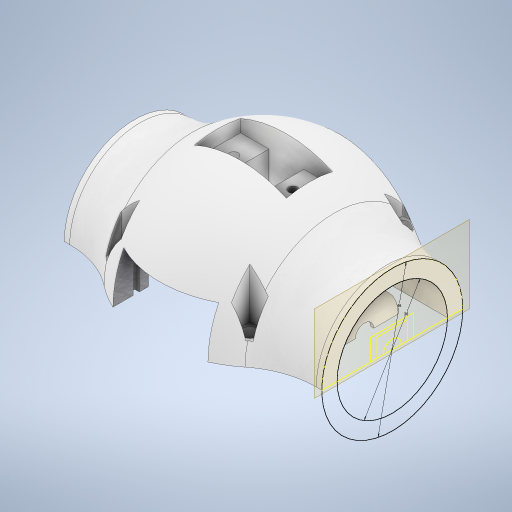
# Autodesk Inventor part: body front moter middle lemon shape
Saved by Autodesk Inventor 2023 (Build 270158000, 158)
## iProperties
Created: 2022-10-08
Part Number: body front moter middle lemon shape
Material: ABS プラスチック
Document SubType Name: Modeling
Designer: ellie
Density: 1.06 g/cm^3
Appearance: 積雪
Author: ellie
Autodesk Inventor part; units mm, degrees
ref_plane "YZ Plane" through (0, 0, 0) normal (1, 0, 0) x (0, 1, 0)
ref_plane "XZ Plane" through (0, 0, 0) normal (0, 1, 0) x (-1, 0, 0)
ref_plane "XY Plane" through (0, 0, 0) normal (0, 0, 1) x (1, 0, 0)
sketch "スケッチ1" plane through (0, 0, 0) normal (0, 1, 0) x (-1, 0, 0)
  circle A0 centre (0, 0) radius 37
  line L0 (0, 0) -> (0, -37)
  line L1 (0, 0) -> (0, 37)
  dimension "d0" = 74
  constraints: 4 end point, 2 point on circle, 2 vertical, 1 centre point, 1 coincident
  measures "d0" diameter of A0
revolve "回転1" add sketch "スケッチ1" angle 180 about axis through (0, 0, 0) along (0, 0, 1) picked at (-2.7444, -24.3574) contours L1 L0 A0
sketch "スケッチ5" plane through (0, 0, 0) normal (0, -1, 0) x (1, 0, 0)
  line L0 (-20, -21) -> (20, -21)
  line L1 (20, -21) -> (20, -11)
  line L2 (20, -11) -> (-20, -11)
  line L3 (-20, -11) -> (-20, -21)
  line L4 (-20, -13) -> (-20, -11)
  line L5 (0, 27) -> (-17, 27)
  line L6 (-17, 27) -> (-17, 25)
  line L7 (-17, 25) -> (0, 25)
  line L8 (0, 25) -> (0, 27)
  line L9 (0, 22) -> (-20, 22)
  line L10 (-20, 22) -> (-20, 21)
  line L11 (-20, 21) -> (0, 21)
  line L12 (0, 21) -> (0, 22)
  line L13 (0, 15) -> (-21, 15)
  line L14 (-21, 15) -> (-21, 13)
  line L15 (-21, 13) -> (0, 13)
  line L16 (0, 13) -> (0, 15)
  line L17 (0, 7) -> (-23, 7)
  line L18 (-23, 7) -> (-23, 5)
  line L19 (-23, 5) -> (0, 5)
  line L20 (0, 5) -> (0, 7)
  circle A0 centre (0, 0) radius 37 projected
  circle A1 centre (0, 0) radius 37 projected
  line L21 (0, 37) -> (0, -37)
  line L22 (37, 0) -> (-37, 0)
  line L23 (-32, 5) -> (-23, 5)
  line L24 (-23, 5) -> (-23, -5)
  line L25 (-23, -5) -> (-32, -5)
  line L26 (-32, -5) -> (-32, 5)
  line L27 (-23, -8.0262) -> (-23, 5)
  line L28 (-29, 22.9783) -> (-29, -22.9783)
  line L29 (-15.5, 27) -> (0, 27)
  line L30 (0, 27) -> (0, 37)
  line L31 (0, 37) -> (-15.5, 37)
  line L32 (-15.5, 37) -> (-15.5, 27)
  line L33 (-15.5, 25) -> (0, 25)
  line L34 (0, 25) -> (0, 22)
  line L35 (0, 22) -> (-15.5, 22)
  line L36 (-15.5, 22) -> (-15.5, 25)
  line L37 (-19, 15) -> (0, 15)
  line L38 (0, 15) -> (0, 21)
  line L39 (0, 21) -> (-19, 21)
  line L40 (-19, 21) -> (-19, 15)
  line L41 (-19, 13) -> (0, 13)
  line L42 (0, 13) -> (0, 7)
  line L43 (0, 7) -> (-19, 7)
  line L44 (-19, 7) -> (-19, 13)
  line L45 (-23, 0) -> (-39.6865, 0)
  line L46 (-23, 0) -> (-7.8337, 0)
  line L47 (-8, 5) -> (-23, 5)
  line L48 (-23, 5) -> (-23, -5)
  line L49 (-23, -5) -> (-8, -5)
  line L50 (-8, -5) -> (-8, 5)
  line L51 (-8, 5) -> (-23, -5) construction
  line L52 (-23, 5) -> (-8, -5) construction
  line L53 (-23, 7) -> (-33, 7)
  line L54 (-33, 7) -> (-33, -7)
  line L55 (-33, -7) -> (-23, -7)
  line L56 (-23, -7) -> (-23, 7)
  line L57 (-23, 7) -> (-33, -7) construction
  line L58 (-33, 7) -> (-23, -7) construction
  line L59 (-8, 5) -> (-1, 5)
  line L60 (-1, 5) -> (-1, -5)
  line L61 (-1, -5) -> (-8, -5)
  line L62 (-8, -5) -> (-8, 5)
  line L63 (-8, 5) -> (-1, -5) construction
  line L64 (-1, 5) -> (-8, -5) construction
  line L65 (-23, 5) -> (-29, 5)
  line L66 (-23, -5) -> (-29, -5)
  line L67 (-23, 7) -> (-29, 7)
  line L68 (-23, -7) -> (-29, -7)
  line L69 (27.2764, -25) -> (-27.2764, -25)
  line L70 (-8, 5) -> (-6.8, 5)
  line L71 (-6.8, 5) -> (-6.8, -5)
  line L72 (-6.8, -5) -> (-8, -5)
  line L73 (-8, -5) -> (-8, 5)
  line L74 (0, 7) -> (2, 7)
  line L75 (0, -3) -> (0, 7)
  line L76 (-11.5791, -11) -> (-8, -11)
  point P0 (0, -21)
  point P1 (0, -11)
  point P2 (0, 26)
  point P3 (0, 21.5)
  point P4 (0, 14)
  point P5 (0, 6)
  point P6 (-20, -16)
  point P7 (-27, -0.5262)
  point P8 (-29, 22.9783)
  point P9 (-29, -22.9783)
  point P10 (-29, -5)
  point P11 (-15.5, 23.5)
  point P12 (-15.5, 33.5969)
  point P13 (0, 27)
  point P14 (0, 37)
  point P15 (0, 25)
  point P16 (0, 13)
  point P17 (0, 15)
  point P18 (-29, 0)
  point P19 (-32, 0)
  point P20 (-23, 0)
  point P21 (-15.5, 0)
  point P22 (-28, 0)
  point P23 (-4.5, 0)
  point P24 (-8, -5)
  point P25 (-8, 5)
  point P26 (-27, 0.5)
  point P27 (-28, 0.4738)
  point P28 (-28, -11.5262)
  point P29 (-27, -11.5)
  point P30 (-23, 5)
  point P31 (-23, 5)
  point P32 (-23, 5)
  point P33 (-8, 0)
  point P34 (-1, 0)
  point P35 (0, 7)
  point P36 (0, 5)
  point P37 (-29, 7)
  dimension "d12" = 40
  dimension "d13" = 10
  dimension "d23" = 17
  dimension "d24" = 2
  dimension "d27" = 20
  dimension "d28" = 1
  dimension "d30" = 21
  dimension "d31" = 2
  dimension "d33" = 2
  dimension "d88" = 0
  dimension "d89" = 0
  dimension "d90" = 16
  dimension "d92" = 20
  dimension "d93" = 10
  dimension "d97" = 9
  dimension "d98" = 10
  dimension "d113" = 29
  dimension "d122" = 15.5
  dimension "d123" = 37
  dimension "d124" = 3
  dimension "d125" = 15.5
  dimension "d126" = 6
  dimension "d127" = 6
  dimension "d147" = 10
  dimension "d149" = 8
  dimension "d151" = 15
  dimension "d161" = 14
  dimension "d162" = 10
  dimension "d164" = 10
  dimension "d165" = 7
  dimension "d170" = 25
  dimension "d175" = 1.2
  dimension "d187" = 1
  dimension "d262" = 2
  dimension "d263" = 2
  constraints: 152 end point, 29 parallel, 19 horizontal, 17 perpendicular, 15 midpoint, 15 point on line, 9 collinear, 1 vertical, 20 other
  measures "d12" distance of L2.end L1.end
  measures "d13" distance of L1.end L0.end
  measures "d23" distance of L7.end L6.end
  measures "d24" distance of L6.end L5.end
  measures "d27" distance of L11.end L10.end
  measures "d28" distance of L10.end L9.end
  measures "d30" distance of L15.end L14.end
  measures "d31" distance of L14.end L13.end
  measures "d33" distance of L18.end L17.end
  measures "d89" distance from line of point (0, 0) L22
  measures "d90" distance from line of L0 point (0, -37)
  measures "d92" distance of the line from the sketch origin of L3
  measures "d93" distance from line of L5 point (0, 37)
  measures "d97" distance of L24.end L25.end
  measures "d98" distance of L23.end L24.end
  measures "d113" distance of the line from the sketch origin of L28
  measures "d122" distance of the line from the sketch origin of L32
  measures "d123" distance between parallel lines of L31 L22
  measures "d124" distance of L33.end L34.end
  measures "d126" distance of L38.end L37.end
  measures "d127" distance of L41.end L42.end
  measures "d147" distance of L48.end L47.end
  measures "d149" distance of the line from the sketch origin of L50
  measures "d151" distance between parallel lines of L50 L24
  measures "d161" distance between parallel lines of L55 L53
  measures "d162" distance between parallel lines of L48 L54
  measures "d164" distance between parallel lines of L61 L59
  measures "d165" distance between parallel lines of L50 L60
  measures "d170" distance between parallel lines of L69 L22
  measures "d175" distance of L71.end L72.end
  measures "d187" distance between parallel lines of L75 L60
  measures "d262" distance between parallel lines of L14 L44
  measures "d263" distance between parallel lines of L14 L40
extrude "GNSボード" cut sketch "スケッチ5" against normal blind 16 contours L8 L7 L6 L5
extrude "GNSボード止めるよう" cut sketch "スケッチ5" against normal blind 15 contours L21 L5 L32 A0 | L21 L9 L36 L7
extrude "アルミ板１" cut sketch "スケッチ5" against normal blind 20 contours L12 L11 L10 L9
extrude "メイン基板" cut sketch "スケッチ5" against normal blind 21 contours L15 L14 L13 L16
extrude "メイン止めるよう" cut sketch "スケッチ5" against normal blind 16.5 contours L17 L44 L15 L21 | L13 L40 L11 L21
extrude "アルミ板２" cut sketch "スケッチ5" against normal blind 20 contours L19 L18 L17 L20
extrude "電池ボックス入れ" cut sketch "スケッチ5" against normal blind 13 contours L3 L2 L21 L0 | L21 L2 L1 L0
extrude "side ut" cut sketch "スケッチ5" against normal blind 100 contours A0 L22 L54 L55 L28 | A0 L28 L53 L54 L22 | L55 L54 L22 L26 L25 L28 | L54 L53 L28 L23 L26 L22 | L25 L26 L22 L28 | L26 L23 L28 L22
extrude "motor case" add sketch "スケッチ5" against normal blind 7 contours L55 L54 L22 L26 L25 L28 | L28 L25 L27 L55 | L54 L53 L28 L23 L26 L22 | L28 L22 L24 L25 | L25 L26 L22 L28 | L53 L18 L23 L28 | L26 L23 L28 L22 | L24 L22 L50 L49 | L28 L23 L24 L22 | L50 L22 L24 L19
extrude "bottom cut" cut sketch "スケッチ5" against normal blind 90 contours L69 A0 L21 | L21 A0 L69
extrude "motor" cut sketch "スケッチ5" against normal blind 6 contours L60 L61 L71 L22 | L22 L71 L19 L60 | L71 L61 L50 L22 | L22 L50 L19 L71 | L28 L22 L24 L25 | L25 L26 L22 L28 | L26 L23 L28 L22 | L24 L22 L50 L49 | L28 L23 L24 L22 | L50 L22 L24 L19
extrude "motor block" add sketch "スケッチ5" against normal blind 10 contours L71 L61 L50 L22 | L22 L50 L19 L71
sketch "スケッチ26" plane through (-33, 0, -7) normal (-1, 0, 0) x (0, 0, 1)
  line L0 (14, 0) -> (0, 0) projected
  circle A0 centre (7, 0) radius 3
  point P0 (7, 0)
  point P1 (7, 0)
  point P2 (7, 0)
  point P3 (7, 0)
  point P4 (4, 0)
  point P5 (10, 0)
  dimension "d197" = 6
  constraints: 1 centre point, 1 coincident
  measures "d197" diameter of A0
extrude "押し出し34" cut sketch "スケッチ26" against normal blind 27 contours L0 A0 picked at (7.7485, 0.6631)
mirror "ミラー11" about plane through (0, 0, 0) normal (1, 0, 0) of "GNSボード", "GNSボード止めるよう", "アルミ板１", "メイン止めるよう", "メイン基板", "アルミ板２", "motor", "押し出し34", "motor case", "電池ボックス入れ", "motor block", "side ut"
ref_plane "作業平面5" through (0, 13, 0) normal (0, -1, 0) x (1, 0, 0)
ref_plane "作業平面6" through (-15.5, 37, 27) normal (0, -1, 0) x (1, 0, 0)
sketch "スケッチ29" plane through (-15.5, 37, 27) normal (0, -1, 0) x (1, 0, 0)
  line L0 (15.5, -27) -> (-67.7134, -27)
  line L1 (-67.7134, -27) -> (15.5, -27)
  line L2 (110.7852, -24.5555) -> (110.7852, -27.3413)
  line L3 (15.5, -27) -> (98.1975, -27)
  circle A0 centre (25.2, -27) radius 1.5
  circle A1 centre (5.8, -27) radius 1.5
  line L4 (32.5, 0) -> (-1.5, 0) projected
  line L5 (15.5, 0) -> (15.5, -52)
  line L6 (-11.7764, -52) -> (42.7764, -52) projected
  point P0 (-11.5, -52)
  point P1 (42.5, -52)
  dimension "d205" = 3
  dimension "d206" = 19.4
  dimension "d207" = 0
  constraints: 10 end point, 2 centre point, 2 horizontal, 2 midpoint, 1 collinear, 1 vertical, 1 other
  measures "d205" diameter of A0
  measures "d206" distance of A1.centre A0.centre
  measures "d207" distance from line of L3 A0.centre
extrude "押し出し36" cut sketch "スケッチ29" along normal blind 25
sketch "スケッチ30" plane through (-15.5, 37, 27) normal (0, -1, 0) x (1, 0, 0)
  line L0 (0.5, -19.5) -> (30.5, -19.5)
  line L1 (30.5, -19.5) -> (30.5, -34.5)
  line L2 (30.5, -34.5) -> (0.5, -34.5)
  line L3 (0.5, -34.5) -> (0.5, -19.5)
  line L4 (0.5, -19.5) -> (30.5, -34.5) construction
  line L5 (30.5, -19.5) -> (0.5, -34.5) construction
  point P0 (15.5, -27)
  dimension "d210" = 30
  dimension "d211" = 15
  constraints: 12 end point, 2 midpoint, 2 parallel, 1 horizontal, 1 perpendicular
  measures "d210" distance of L1.end L2.end
  measures "d211" distance of L0.end L1.end
extrude "押し出し37" cut sketch "スケッチ30" along normal blind 8
ref_plane "作業平面7" through (-15.5, 12, 27) normal (0, 1, 0) x (1, 0, 0)
sketch "スケッチ33" plane through (-15.5, 12, 27) normal (0, 1, 0) x (1, 0, 0)
  circle A0 centre (25.2, 27) radius 1.5 projected
  circle A1 centre (5.8, 27) radius 1.5 projected
  line L0 (0.5, 34.5) -> (0.5, 19.5) projected
  line L1 (30.5, 19.5) -> (30.5, 34.5) projected
  line L2 (0.5, 19.5) -> (30.5, 19.5) projected
  line L3 (30.5, 34.5) -> (0.5, 34.5) projected
  line L4 (15.5, 0) -> (15.5, 52) projected
  line L5 (15.5, 27) -> (98.1975, 27) projected
  circle A2 centre (25.2, 27) radius 3
  circle A3 centre (5.8, 27) radius 3
  dimension "d219" = 6
  dimension "d220" = 6
  constraints: 2 centre point, 2 coincident
  measures "d219" diameter of A2
  measures "d220" diameter of A3
extrude "押し出し39" cut sketch "スケッチ33" along normal blind 10 contours L5 A0 | L5 A2 A0 | A0 L5 A2 | A0 L5 | A1 | A3
sketch "スケッチ35" plane through (-17, 0, 25) normal (0, -1, 0) x (1, 0, 0)
  circle A0 centre (-4, 0.4) radius 2.4
  line L0 (9, -30) -> (9, -20) projected
  line L1 (-6, -20) -> (9, -20) projected
  line L2 (-15, -20) -> (-6, -20) projected
  line L3 (-15, -30) -> (-15, -20) projected
  line L4 (16, -30) -> (10.2, -30) projected
  line L5 (-16, -22) -> (-15, -22) projected
  line L6 (-15, -22) -> (-15, -20) projected
  line L7 (-15, -20) -> (-6, -20) projected
  line L8 (-6, -20) -> (-6, -18) projected
  line L9 (-6, -18) -> (-2, -18) projected
  line L10 (-2, -18) -> (-2, -12) projected
  line L11 (-2, -12) -> (-4, -12) projected
  line L12 (-4, -12) -> (-4, -10) projected
  line L13 (-4, -10) -> (-2, -10) projected
  line L14 (-2, -10) -> (-2, -4) projected
  line L15 (-2, -4) -> (-3, -4) projected
  line L16 (-3, -4) -> (-3, -3) projected
  line L17 (-3, -3) -> (1.5, -3) projected
  line L18 (1.5, -3) -> (1.5, 0) projected
  line L19 (1.5, 0) -> (0, 0) projected
  line L20 (0, 0) -> (0, 2) projected
  line L21 (0, 2) -> (1.5, 2) projected
  line L22 (1.5, 2) -> (1.5, 8.5969) projected
  arc A1 (1.5, 8.5969) -> (-12, -2.0217) centre (17, -25) ccw projected
  line L23 (-12, -2.0217) -> (-12, -18) projected
  line L24 (-12, -18) -> (-16, -18) projected
  line L25 (-16, -18) -> (-16, -22) projected
  line L26 (10.2, -20) -> (10.2, -30) projected
  line L27 (16, -20) -> (16, -30) projected
  line L28 (10.2, -20) -> (16, -20) projected
  line L29 (9, -30) -> (-15, -30) projected
  point P0 (-15, -22)
  dimension "d231" = 4.8
  dimension "d233" = 1
  dimension "d234" = 4
  constraints: 1 centre point
  measures "d231" diameter of A0
  measures "d233" distance edge to line of A0 L17
  measures "d234" distance from line of A0.centre L20
extrude "押し出し41" cut sketch "スケッチ35" against normal blind 20 contours A0
mirror "ミラー12" about plane through (0, 0, 0) normal (1, 0, 0) of "押し出し41"
sketch "スケッチ36" plane through (-33, 0, -7) normal (0, -1, 0) x (1, 0, 0)
  circle A0 centre (9, -14.5) radius 2.4
  line L0 (41, 4) -> (39.8, 4) projected
  line L1 (39.8, 2) -> (39.8, 4) projected
  line L2 (34, 2) -> (34, 12) projected
  line L3 (34, 12) -> (32, 12) projected
  line L4 (32, 12) -> (32, 2) projected
  line L5 (26.2, 2) -> (26.2, 4) projected
  line L6 (26.2, 4) -> (25, 4) projected
  line L7 (25, 12) -> (25, 10) projected
  line L8 (10, 12) -> (10, 14) projected
  line L9 (32, 2) -> (26.2, 2) projected
  line L10 (1, 2) -> (1, 4) projected
  line L11 (1, 4) -> (0, 4) projected
  line L12 (0, 4) -> (0, 0) projected
  line L13 (0, 0) -> (4, 0) projected
  line L14 (4, 0) -> (4, -15.9783) projected
  arc A1 (4, -15.9783) -> (5.7236, -18) centre (33, 7) ccw projected
  line L15 (5.7236, -18) -> (60.2764, -18) projected
  arc A2 (60.2764, -18) -> (62, -15.9783) centre (33, 7) ccw projected
  line L16 (62, -15.9783) -> (62, 0) projected
  line L17 (66, 0) -> (62, 0) projected
  line L18 (66, 4) -> (66, 0) projected
  line L19 (66, 4) -> (65, 4) projected
  line L20 (65, 4) -> (65, 2) projected
  line L21 (39.8, 2) -> (34, 2) projected
  line L22 (56, 14) -> (56, 12) projected
  line L23 (41, 12) -> (41, 10) projected
  line L24 (13, -4) -> (53, -4) projected
  line L25 (53, -4) -> (53, -14) projected
  line L26 (53, -14) -> (13, -14) projected
  line L27 (13, -14) -> (13, -4) projected
  line L28 (53, -4) -> (53, -14) projected
  line L29 (13, -4) -> (53, -4) projected
  line L30 (13, -14) -> (13, -4) projected
  line L31 (53, -14) -> (13, -14) projected
  line L32 (0, 10) -> (1, 10) projected
  line L33 (1, 10) -> (1, 12) projected
  line L34 (1, 12) -> (10, 12) projected
  line L35 (10, 14) -> (14, 14) projected
  line L36 (14, 14) -> (14, 20) projected
  line L37 (14, 20) -> (12, 20) projected
  line L38 (12, 20) -> (12, 22) projected
  line L39 (12, 22) -> (14, 22) projected
  line L40 (14, 22) -> (14, 28) projected
  line L41 (14, 28) -> (13, 28) projected
  line L42 (13, 28) -> (13, 29) projected
  line L43 (13, 29) -> (17.5, 29) projected
  line L44 (17.5, 29) -> (17.5, 32) projected
  line L45 (17.5, 32) -> (16, 32) projected
  line L46 (16, 32) -> (16, 34) projected
  line L47 (16, 34) -> (17.5, 34) projected
  line L48 (17.5, 34) -> (17.5, 40.5969) projected
  line L49 (4, 29.9783) -> (4, 14) projected
  line L50 (4, 14) -> (0, 14) projected
  line L51 (0, 14) -> (0, 10) projected
  line L52 (25, 10) -> (26.2, 10) projected
  line L53 (26.2, 10) -> (26.2, 12) projected
  line L54 (26.2, 12) -> (25, 12) projected
  line L55 (25, 4) -> (25, 2) projected
  line L56 (25, 2) -> (1, 2) projected
  line L57 (65, 2) -> (41, 2) projected
  line L58 (41, 4) -> (41, 2) projected
  line L59 (39.8, 10) -> (41, 10) projected
  line L60 (39.8, 12) -> (41, 12) projected
  line L61 (39.8, 10) -> (39.8, 12) projected
  line L62 (65, 10) -> (66, 10) projected
  line L63 (66, 14) -> (66, 10) projected
  line L64 (62, 14) -> (66, 14) projected
  line L65 (62, 14) -> (62, 29.9783) projected
  line L66 (48.5, 40.5969) -> (48.5, 34) projected
  line L67 (48.5, 34) -> (50, 34) projected
  line L68 (50, 34) -> (50, 32) projected
  line L69 (50, 32) -> (48.5, 32) projected
  line L70 (48.5, 32) -> (48.5, 29) projected
  line L71 (48.5, 29) -> (53, 29) projected
  line L72 (53, 29) -> (53, 28) projected
  line L73 (53, 28) -> (52, 28) projected
  line L74 (52, 28) -> (52, 22) projected
  line L75 (52, 22) -> (54, 22) projected
  line L76 (54, 22) -> (54, 20) projected
  line L77 (54, 20) -> (52, 20) projected
  line L78 (52, 20) -> (52, 14) projected
  line L79 (52, 14) -> (56, 14) projected
  line L80 (56, 12) -> (65, 12) projected
  line L81 (65, 12) -> (65, 10) projected
  circle A3 centre (12, 32.4) radius 2.4 projected
  circle A4 centre (54, 32.4) radius 2.4 projected
  arc A5 (17.5, 40.5969) -> (4, 29.9783) centre (33, 7) ccw projected
  arc A6 (62, 29.9783) -> (48.5, 40.5969) centre (33, 7) ccw projected
  dimension "d237" = 4.8
  dimension "d238" = 4
  dimension "d239" = 16.5
  constraints: 1 centre point
  measures "d237" diameter of A0
  measures "d238" distance from line of A0.centre L27
  measures "d239" distance from line of A0.centre L9
extrude "押し出し42" cut sketch "スケッチ36" against normal blind 25 contours A0
mirror "ミラー13" about plane through (0, 0, 0) normal (1, 0, 0) of "押し出し42"
ref_plane "作業平面8" through (-17, 35, 25) normal (0, -1, 0) x (1, 0, 0)
sketch "スケッチ37" plane through (-17, 35, 25) normal (0, -1, 0) x (1, 0, 0)
  line L0 (38, -10) -> (-4, -10) projected
  line L1 (2, -17.5) -> (2, -32.5) projected
  line L2 (32, -32.5) -> (32, -17.5) projected
  arc A0 (32.5, 5.0624) -> (1.5, 5.0624) centre (17, -25) ccw projected
  line L3 (32.5, 5.0624) -> (32.5, 8.5969) projected
  line L4 (46, -2.0217) -> (46, -47.9783) projected
  arc A1 (44.2764, -50) -> (46, -47.9783) centre (17, -25) ccw projected
  line L5 (44.2764, -50) -> (-10.2764, -50) projected
  arc A2 (-12, -47.9783) -> (-10.2764, -50) centre (17, -25) ccw projected
  line L6 (-12, -47.9783) -> (-12, -2.0217) projected
  line L7 (1.5, 8.5969) -> (1.5, 5.0624) projected
  line L8 (-7, 3.4) -> (-1, 3.4)
  line L9 (-1, 3.4) -> (-1, -2.6)
  line L10 (-1, -2.6) -> (-7, -2.6)
  line L11 (-7, -2.6) -> (-7, 3.4)
  arc A3 (37.6, -40) -> (37.6, -40) centre (-4, 0.4) ccw projected
  line L12 (-7, 3.4) -> (-1, -2.6) construction
  line L13 (-1, 3.4) -> (-7, -2.6) construction
  line L14 (41, 3.4) -> (35, 3.4)
  line L15 (35, 3.4) -> (35, -2.6)
  line L16 (35, -2.6) -> (41, -2.6)
  line L17 (41, -2.6) -> (41, 3.4)
  arc A4 (37.6, -40) -> (37.6, -40) centre (38, 0.4) ccw projected
  line L18 (41, 3.4) -> (35, -2.6) construction
  line L19 (35, 3.4) -> (41, -2.6) construction
  line L20 (-4, -43.5) -> (-10, -43.5)
  line L21 (-10, -43.5) -> (-10, -49.5)
  line L22 (-10, -49.5) -> (-4, -49.5)
  line L23 (-4, -49.5) -> (-4, -43.5)
  circle A5 centre (-7, -46.5) radius 2.4 projected
  line L24 (-4, -43.5) -> (-10, -49.5) construction
  line L25 (-10, -43.5) -> (-4, -49.5) construction
  line L26 (44, -43.5) -> (38, -43.5)
  line L27 (38, -43.5) -> (38, -49.5)
  line L28 (38, -49.5) -> (44, -49.5)
  line L29 (44, -49.5) -> (44, -43.5)
  circle A6 centre (41, -46.5) radius 2.4 projected
  line L30 (44, -43.5) -> (38, -49.5) construction
  line L31 (38, -43.5) -> (44, -49.5) construction
  line L32 (32, -17.5) -> (2, -17.5) projected
  line L33 (2, -32.5) -> (32, -32.5) projected
  arc A7 (46, -2.0217) -> (32.5, 8.5969) centre (17, -25) ccw projected
  arc A8 (1.5, 8.5969) -> (-12, -2.0217) centre (17, -25) ccw projected
  point P0 (-1.6, 0.4)
  point P1 (35.6, 0.4)
  point P2 (-3.6, -40)
  point P3 (36.5, 1.5)
  point P4 (-2.5, 1.5)
  dimension "d243" = 6
  dimension "d244" = 6
  dimension "d245" = 6
  dimension "d246" = 6
  dimension "d247" = 6
  dimension "d248" = 6
  dimension "d249" = 6
  dimension "d250" = 6
  constraints: 48 end point, 8 midpoint, 8 parallel, 4 horizontal, 4 perpendicular, 10 other
  measures "d243" distance of L9.end L10.end
  measures "d244" distance of L8.end L9.end
  measures "d245" distance of L16.end L15.end
  measures "d246" distance of L15.end L14.end
  measures "d247" distance of L22.end L21.end
  measures "d248" distance of L21.end L20.end
  measures "d249" distance of L28.end L27.end
  measures "d250" distance of L27.end L26.end
extrude "押し出し43" cut sketch "スケッチ37" along normal blind 20 contours L23 L22 L21 L20 | A5 | L29 L28 L27 L26 | A6
extrude "押し出し44" cut sketch "スケッチ37" along normal blind 28 contours A4 L8 L9 L10 | L10 L11 A8 L8 A4 | L11 L8 A8 | A7 L14 L17 | L17 L16 L15 L14 A7
sketch "スケッチ39" plane through (-15.5, 29, 27) normal (0, 1, 0) x (1, 0, 0)
  line L0 (21.2, 19.5) -> (9.8, 19.5)
  line L1 (9.8, 19.5) -> (9.8, 34.5)
  line L2 (9.8, 34.5) -> (21.2, 34.5)
  line L3 (21.2, 34.5) -> (21.2, 19.5)
  line L4 (21.2, 19.5) -> (9.8, 34.5) construction
  line L5 (9.8, 19.5) -> (21.2, 34.5) construction
  circle A0 centre (5.8, 27) radius 1.5 projected
  circle A1 centre (25.2, 27) radius 1.5 projected
  line L6 (0.5, 19.5) -> (30.5, 19.5) projected
  line L7 (30.5, 34.5) -> (0.5, 34.5) projected
  circle A2 centre (5.8, 27) radius 1.5 projected
  circle A3 centre (25.2, 27) radius 1.5 projected
  line L8 (0.5, 34.5) -> (30.5, 34.5) projected
  line L9 (0.5, 19.5) -> (0.5, 34.5) projected
  line L10 (30.5, 19.5) -> (0.5, 19.5) projected
  line L11 (30.5, 34.5) -> (30.5, 19.5) projected
  point P0 (15.5, 27)
  dimension "d255" = 4
  dimension "d256" = 0
  constraints: 12 end point, 2 midpoint, 2 parallel, 1 horizontal, 1 perpendicular
  measures "d255" distance from line of L1 A0.centre
  measures "d256" distance between parallel lines of L6 L0
extrude "押し出し45" cut sketch "スケッチ39" against normal up to surface (12.5 mm away) contours L0 L1 L2 L3
ref_plane "作業平面9" through (42, 0, -7) normal (1, 0, 0) x (0, 0, -1)
sketch "スケッチ41" plane through (42, 0, -7) normal (1, 0, 0) x (0, 0, -1)
  arc A0 (-4, 0) -> (-10, 0) centre (-7, 0) ccw projected
  arc A1 (-4, 0) -> (-10, 0) centre (-7, 0) ccw projected
  line L0 (-4, 0) -> (0, 0) projected
  line L1 (0, 0) -> (0, 7) projected
  line L2 (0, 7) -> (-14, 7) projected
  line L3 (-14, 0) -> (-14, 7) projected
  line L4 (-14, 0) -> (-10, 0) projected
  line L5 (0, 7) -> (0, 0) projected
  line L6 (15.9783, 0) -> (0, 0) projected
  arc A2 (15.9783, 0) -> (-29.9783, 0) centre (-7, 0) ccw projected
  line L7 (-14, 0) -> (-29.9783, 0) projected
  line L8 (-14, 0) -> (-14, 7) projected
  line L9 (-14, 7) -> (0, 7) projected
  line L10 (-2, 0) -> (-12, 0) projected
  line L11 (-2, 0) -> (-2, 6) projected
  line L12 (-12, 6) -> (-2, 6) projected
  line L13 (-12, 0) -> (-12, 6) projected
  circle A3 centre (-7, 0) radius 23
  circle A4 centre (-7, 0) radius 18
  point P0 (-25, 0)
  point P1 (11, 0)
  dimension "d267" = 46
  dimension "d268" = 36
  constraints: 2 centre point, 2 coincident
  measures "d267" diameter of A3
  measures "d268" diameter of A4
extrude "押し出し47" add sketch "スケッチ41" against normal up to surface (13 mm away) contours A4 L7 A2 L6
fillet "面フィレット1" radius 27.7 1 edges at (29, 22.9783, 0)
mirror "ミラー14" about plane through (0, 0, 0) normal (1, 0, 0) of "面フィレット1", "押し出し47"
sketch "スケッチ42" plane through (0, 16.5, 0) normal (0, -1, 0) x (1, 0, 0)
  line L0 (-5.7, 7.5) -> (5.7, 7.5) projected
  line L1 (-5.7, 5) -> (-5.7, 7) projected
  line L2 (5.7, 7) -> (5.7, 5) projected
  line L3 (15, 7.5) -> (5.7, 7.5) projected
  line L4 (5.7, 7.5) -> (-5.7, 7.5)
  line L5 (-5.7, 7.5) -> (-5.7, 10.5)
  line L6 (-5.7, 10.5) -> (5.7, 10.5)
  line L7 (5.7, 10.5) -> (5.7, 7.5)
  point P0 (0, 0)
  dimension "d272" = 3
  constraints: 8 end point, 3 parallel, 1 horizontal, 1 perpendicular
  measures "d272" distance of L6.end L0.end
extrude "押し出し48" cut sketch "スケッチ42" against normal blind 10
sketch "スケッチ43" plane through (33, 0, -3) normal (1, 0, 0) x (0, 0, -1)
  arc A0 (0, 0) -> (-6, 0) centre (-3, 0) ccw projected
  circle A1 centre (-3, 0) radius 11
  arc A2 (15, 0) -> (-21, 0) centre (-3, 0) ccw projected
  line L0 (-10, 0) -> (-21, 0) projected
  line L1 (-10, 0) -> (-10, 7) projected
  line L2 (-10, 7) -> (4, 7) projected
  line L3 (4, 7) -> (4, 0) projected
  line L4 (15, 0) -> (4, 0) projected
  line L5 (-10, 0) -> (-6, 0) projected
  line L6 (0, 0) -> (4, 0) projected
  line L7 (2, 0) -> (-8, 0) projected
  point P0 (-3, 0)
  point P1 (8, 0)
  point P2 (-14, 0)
  dimension "d275" = 22
  constraints: 1 centre point, 1 coincident
  measures "d275" diameter of A1
extrude "押し出し49" add sketch "スケッチ43" against normal up to surface (4 mm away) contours L3 L2 L1 L0 A1 L4
mirror "ミラー15" about plane through (0, 0, 0) normal (1, 0, 0) of "押し出し49"
sketch "スケッチ44" plane through (-33, 0, 0) normal (-1, 0, 0) x (0, 0, 1)
  point P0 (0, 0)
sketch "スケッチ45" plane through (-29, 0, 0) normal (-1, 0, 0) x (0, 0, 1)
  circle A0 centre (0, 0) radius 11
  arc A1 (3, 0) -> (-3, 0) centre (0, 0) ccw projected
  circle A2 centre (0, 0) radius 18
  line L0 (18, 0) -> (11, 0) projected
  line L1 (-11, 0) -> (-18, 0) projected
  dimension "d278" = 22
  dimension "d279" = 36
  constraints: 2 centre point, 2 coincident
  measures "d278" diameter of A0
  measures "d279" diameter of A2
extrude "押し出し50" cut sketch "スケッチ45" against normal blind 5 contours A0 L1 A2 L0 picked at (-15.4923, 1.4359)
mirror "ミラー16" about plane through (0, 0, 0) normal (1, 0, 0) of "押し出し50"
